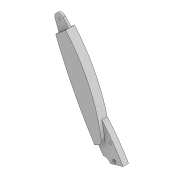
# Autodesk Inventor part: zijkant
Saved by Autodesk Inventor 2020.3 (Build 243373000, 373)
## iProperties
Created: 2020-09-15
Part Number: zijkant
Material: Generic
Document SubType Name: Modeling
Designer: Svend
Density: 1 g/cm^3
Appearance: Default
Author: Svend
Autodesk Inventor part; units mm, degrees
ref_plane "YZ Plane" through (0, 0, 0) normal (1, 0, 0) x (0, 1, 0)
ref_plane "XZ Plane" through (0, 0, 0) normal (0, 1, 0) x (-1, 0, 0)
ref_plane "XY Plane" through (0, 0, 0) normal (0, 0, 1) x (1, 0, 0)
ref_plane "Work Plane1" through (0, 0, 0) normal (0, 0, 1) x (1, 0, 0)
sketch "Sketch1" plane through (0, 0, 0) normal (0, 0, 1) x (1, 0, 0)
  circle A0 centre (70, 0) radius 5 projected
  circle A1 centre (293.8763, -377.7839) radius 4.188 projected
  circle A2 centre (293.8763, -377.7839) radius 8.8 projected
  arc A3 (63.7, -21.6) -> (-63.7, -21.6) centre (0, -240) ccw projected
  arc A4 (63.7, -21.6) -> (63.7, 21.6) centre (70, 0) ccw projected
  arc A5 (-63.7, 21.6) -> (63.7, 21.6) centre (0, 240) ccw projected
  arc A6 (-63.7, 21.6) -> (-63.7, -21.6) centre (-70, 0) ccw projected
  circle A7 centre (70, 0) radius 5 projected
  circle A8 centre (-70, 0) radius 5 projected
  arc A9 (103.2014, -50.6129) -> (104.1376, -47.9439) centre (102.335, -48.8103) ccw projected
  line L0 (104.1376, -47.9439) -> (88.9974, -16.4423) projected
  arc A10 (89.2305, -11.6806) -> (88.9974, -16.4423) centre (93.504, -14.2763) ccw projected
  arc A11 (89.2305, -11.6806) -> (67.1075, -22.3133) centre (70, 0) ccw projected
  arc A12 (70.9713, -25.1059) -> (67.1075, -22.3133) centre (66.4648, -27.2718) ccw projected
  line L1 (70.9713, -25.1059) -> (86.1115, -56.6076) projected
  arc A13 (86.1115, -56.6076) -> (88.7805, -57.5438) centre (87.9141, -55.7412) ccw projected
  line L2 (88.7805, -57.5438) -> (103.2014, -50.6129) projected
  circle A14 centre (70, 0) radius 5 projected
  circle A15 centre (90.3596, -42.3614) radius 3 projected
  line L3 (49.0525, -8.2129) -> (67.0441, -54.1018)
  line L4 (67.0441, -54.1018) -> (112.5529, -15)
  line L5 (112.5529, -15) -> (87.0658, 14.6632)
  point P0 (0, 0)
  point P1 (87.0658, 14.6632)
  dimension "d0" = 15
  dimension "d1" = 15
  dimension "d2" = 60
  dimension "d3" = 15
  constraints: 6 end point, 2 point on circle, 2 tangent
  measures "d0" angle of L4 L2
  measures "d1" angle of L0 L5
  measures "d2" distance of L3.end L4.end
  measures "d3" vertical distance of L4.end A0.centre
extrude "Extrusion1" add sketch "Sketch1" along normal blind 10 contours A4 A12 L1 L4 L3 A3 | A11 A4 | A3 L3 A11 | A4 A10 L0 L4 L1 A12 | A4 L5 L4 L0 A10
ref_plane "Work Plane2" through (70, 0, 10) normal (0.7584791, 0.6516974, 0) x (0, 0, -1)
ref_plane "Work Plane3" through (0, 0, 5) normal (0, 0, -1) x (-1, 0, 0)
sketch "Sketch2" plane through (0, 0, 5) normal (0, 0, -1) x (-1, 0, 0)
  line L0 (-112.5529, -15) -> (-87.0658, 14.6632) projected
  arc A0 (-49.0525, -8.2129) -> (-87.0658, 14.6632) centre (-70, 0) ccw projected
  line L1 (-49.0525, -8.2129) -> (-67.0441, -54.1018) projected
  line L2 (-67.0441, -54.1018) -> (-112.5529, -15) projected
  circle A1 centre (-70, 0) radius 5 projected
  arc A2 (-244.1237, -401.5825) -> (-67.0441, -54.1018) centre (-1929.046, 675.9317) ccw
  line L3 (-112.5529, -15) -> (-87.0658, 14.6632) projected
  arc A3 (-112.5529, -15) -> (-278.7081, -396.2045) centre (423.2088, -475.3351) ccw
  line L4 (-244.1237, -401.5825) -> (-309.4333, -366.064)
  point P0 (0, 0)
  point P1 (-259.1297, -424.6952)
  point P2 (-274.6513, -366.064)
  point P3 (-277.1734, -383.6085)
  dimension "d8" = 390
  dimension "d9" = 2000
  dimension "d11" = 35
  constraints: 6 point on circle, 2 centre point, 2 end point, 2 tangent
  measures "d8" distance of L1.end L4.start
  measures "d9" radius of A2
  measures "d11" distance of L4.start A3.end
extrude "Extrusion2" add sketch "Sketch2" along normal mid plane 40 contours L2 A2 L4 A3
fillet "Fillet1" radius 20 1 edges at (277.1734, -383.6085, 5)
sketch "Sketch3" plane through (0, 0, -15) normal (0, 0, -1) x (-1, 0, 0)
  line L0 (-67.0441, -54.1018) -> (-112.5529, -15) projected
  line L1 (-81.9461, -41.2978) -> (-96.952, -72.52)
  line L2 (-96.952, -72.52) -> (-114.9782, -63.8563)
  line L3 (-114.9782, -63.8563) -> (-97.6509, -27.8041)
  line L4 (-105.9651, -68.1881) -> (-89.7985, -34.5509) construction
  point P0 (0, 0)
  dimension "d20" = 75
  dimension "d21" = 40
  dimension "d22" = 20
  constraints: 8 end point, 3 perpendicular, 2 midpoint, 2 point on line
  measures "d20" angle of L0 L1
  measures "d21" distance from line of L3.end L2
  measures "d22" distance between parallel lines of L3 L1
extrude "Extrusion3" cut sketch "Sketch3" against normal up to surface (15 mm away)
fillet "Fillet3" radius 5 2 edges at (114.9782, -63.8563, -7.5) (96.952, -72.52, -7.5)
ref_plane "Work Plane4" through (0, 0, 10) normal (0, 0, 1) x (1, 0, 0)
sketch "Sketch4" plane through (0, 0, 10) normal (0, 0, 1) x (1, 0, 0)
  arc A0 (275.2071, -369.6744) -> (112.5529, -15) centre (-423.2088, -475.3351) ccw projected
  line L0 (112.5529, -15) -> (67.0441, -54.1018) projected
  arc A1 (67.0441, -54.1018) -> (244.1237, -401.5825) centre (1929.046, 675.9317) ccw projected
  arc A2 (244.1237, -401.5825) -> (268.7928, -439.2181) centre (1929.046, 675.9317) ccw
  arc A3 (277.1734, -383.6085) -> (112.5529, -15) centre (-423.2088, -475.3351) ccw projected
  arc A4 (358.7663, -437.0377) -> (261.451, -301.5825) centre (-417.6707, -892.1702) ccw
  line L1 (268.7928, -439.2181) -> (358.7663, -437.0377) construction
  line L2 (358.7663, -437.0377) -> (301.204, -453.9664)
  arc A5 (301.204, -453.9664) -> (268.7928, -439.2181) centre (274.998, -468.5693) ccw
  line L3 (244.1237, -401.5825) -> (264.9874, -390.2358) projected
  arc A6 (264.9874, -390.2358) -> (275.2071, -369.6744) centre (255.4321, -372.6661) ccw projected
  point P0 (0, 0)
  point P1 (290.4905, -391.477)
  point P2 (261.451, -301.5825)
  point P3 (275.2071, -369.6744)
  dimension "d25" = 45
  dimension "d27" = 120
  dimension "d29" = 900
  dimension "d33" = 90
  dimension "d34" = 30
  dimension "d35" = 60
  dimension "d36" = 15
  dimension "d39" = 100
  constraints: 8 point on circle, 4 end point, 3 centre point, 2 concentric
  measures "d25" distance of L3.start L1.start
  measures "d27" distance of L3.start L1.end
  measures "d29" radius of A4
  measures "d33" distance of L1.start L1.end
  measures "d34" radius of A5
  measures "d35" distance of L1.end L2.end
  measures "d36" angle of L2 L1
  measures "d39" vertical distance of L3.start A4.end
extrude "Extrusion4" add sketch "Sketch4" against normal up to surface (25 mm away) contours A0 A4 L2 A5 A2 L3 A6
sketch "Sketch5" plane through (0, 0, 10) normal (0, 0, 1) x (1, 0, 0)
  circle A0 centre (70, 0) radius 5 projected
  arc A1 (358.7663, -437.0377) -> (261.451, -301.5825) centre (-417.6707, -892.1702) ccw projected
  arc A2 (275.2071, -369.6744) -> (261.451, -301.5825) centre (-423.2088, -475.3351) ccw projected
  arc A3 (264.9874, -390.2358) -> (275.2071, -369.6744) centre (255.4321, -372.6661) ccw projected
  line L0 (244.1237, -401.5825) -> (264.9874, -390.2358) projected
  arc A4 (244.1237, -401.5825) -> (268.7928, -439.2181) centre (1929.046, 675.9317) ccw projected
  arc A5 (301.204, -453.9664) -> (268.7928, -439.2181) centre (274.998, -468.5693) ccw projected
  line L1 (301.204, -453.9664) -> (358.7663, -437.0377) projected
  circle A6 centre (300.6543, -373.6842) radius 5
  line L2 (300.6543, -373.6842) -> (70, 0) construction
  circle A7 centre (318.9937, -436.0434) radius 7.5
  line L3 (318.9937, -436.0434) -> (300.6543, -373.6842) construction
  point P0 (0, 0)
  dimension "d40" = 10
  dimension "d41" = 439.137
  dimension "d43" = 2.5
  dimension "d44" = 15
  dimension "d45" = 65
  dimension "d46" = 90
  constraints: 4 end point, 2 centre point
  measures "d40" diameter of A6
  measures "d41" distance of L2.start L2.end
  measures "d43" distance from line of L0 L2.start
  measures "d44" diameter of A7
  measures "d45" distance of L3.start L2.start
  measures "d46" angle of L1 L3
extrude "Extrusion5" cut sketch "Sketch5" against normal through all contours A6
extrude "Extrusion6" cut sketch "Sketch5" against normal blind 20 contours A7
body "Solid1"
